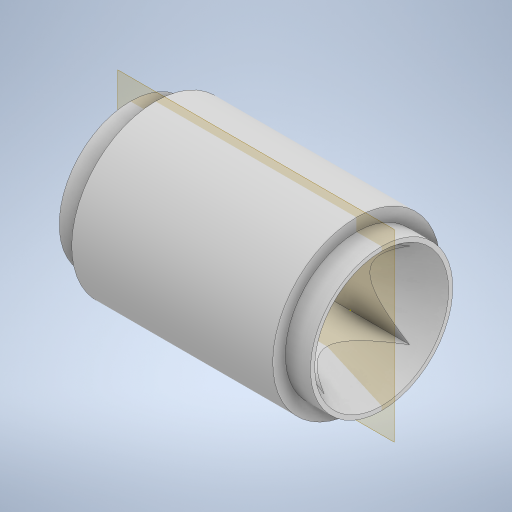
# Autodesk Inventor part: Bartosz_Zukowski_model_nr_13
Saved by Autodesk Inventor 2024 (Build 280153000, 153)
## iProperties
Created: 2024-04-24
Part Number: Bartosz_Zukowski_model_nr_13
Material: Ogólny
Document SubType Name: Modeling
Designer: student156p
Density: 1 g/cm^3
Appearance: Domyślna
Author: student156p
Autodesk Inventor part; units mm, degrees
ref_plane "YZ Plane" through (0, 0, 0) normal (1, 0, 0) x (0, 1, 0)
ref_plane "XZ Plane" through (0, 0, 0) normal (0, 1, 0) x (-1, 0, 0)
sketch "Szkic1" plane through (0, 0, 0) normal (0, 0, 1) x (1, 0, 0)
  point P0 (0, 0)
sketch "Szkic2" plane through (0, 0, 0) normal (0, 0, 1) x (1, 0, 0)
  line L0 (-26.25, 0) -> (-26.25, 8.5)
  line L1 (-26.25, 8.5) -> (-23.25, 8.5)
  line L2 (-23.25, 8.5) -> (-23.25, 10)
  line L3 (-23.25, 10) -> (0.75, 10)
  line L4 (0.75, 10) -> (0.75, 8.5)
  line L5 (0.75, 8.5) -> (3.75, 8.5)
  line L6 (3.75, 8.5) -> (3.75, 0)
  line L7 (3.75, 0) -> (-26.25, 0)
  point P0 (0, 0)
  dimension "d0" = 30
  dimension "d2" = 3
  dimension "d3" = 24
  dimension "d4" = 20
  dimension "d5" = 17
  constraints: 16 end point, 3 perpendicular, 1 collinear, 1 vertical
  measures "d0" distance between parallel lines of L6 L0
  measures "d2" distance between parallel lines of L2 L0
  measures "d3" distance between parallel lines of L4 L2
  measures "d4" diameter of L3 L7
  measures "d5" diameter of L5 L7
revolve "Obrót1" add sketch "Szkic2" angle 360 about axis through (3.75, 0, 0) along (-1, 0, 0)
sketch "Szkic3" plane through (3.75, 0, 0) normal (1, 0, 0) x (0, 0, -1)
  circle A0 centre (0, 0) radius 8
  dimension "d7" = 16
  constraints: 1 centre point, 1 coincident
  measures "d7" diameter of A0
extrude "Wyciągnięcie proste1" cut sketch "Szkic3" against normal blind 10 draft -24
sketch "Szkic4" plane through (-26.25, 0, 0) normal (-1, 0, 0) x (0, 0, 1)
  line L0 (-5.1, -5.1) -> (5.1, -5.1)
  line L1 (5.1, -5.1) -> (5.1, 5.1)
  line L2 (5.1, 5.1) -> (-5.1, 5.1)
  line L3 (-5.1, 5.1) -> (-5.1, -5.1)
  line L4 (-5.1, -5.1) -> (5.1, 5.1) construction
  line L5 (5.1, -5.1) -> (-5.1, 5.1) construction
  point P0 (0, 0)
  dimension "d10" = 10.2
  dimension "d11" = 10.2
  constraints: 12 end point, 2 midpoint, 2 parallel, 1 horizontal, 1 perpendicular
  measures "d10" distance of L2.end L1.end
  measures "d11" distance of L1.end L0.end
extrude "Wyciągnięcie proste2" cut sketch "Szkic4" against normal through all
sketch "Szkic5" plane through (-26.25, 0, 0) normal (-1, 0, 0) x (0, 0, 1)
  circle A0 centre (0, 0) radius 8
  dimension "d14" = 16
  constraints: 1 centre point, 1 coincident
  measures "d14" diameter of A0
extrude "Wyciągnięcie proste3" cut sketch "Szkic5" against normal blind 10 draft -24
sketch "Szkic6" plane through (0, 0, 0) normal (0, 0, 1) x (1, 0, 0)
  point P0 (0, 0)
